Autodesk Fusion 360 part; units mm, degrees
(part 2 of 40)
  line L405 (261.8534, 192.3041) -> (262.0044, 192.3574) construction
  line L406 (262.0044, 192.3574) -> (262.156, 192.4097) construction
  line L407 (262.156, 192.4097) -> (262.3081, 192.461) construction
  line L408 (262.3081, 192.461) -> (262.4608, 192.5114) construction
  line L409 (262.4608, 192.5114) -> (262.614, 192.5608) construction
  line L410 (262.614, 192.5608) -> (262.7678, 192.6094) construction
  line L411 (262.7678, 192.6094) -> (262.922, 192.657) construction
  line L412 (262.922, 192.657) -> (263.0767, 192.7037) construction
  line L413 (263.0767, 192.7037) -> (263.2319, 192.7495) construction
  line L414 (263.2319, 192.7495) -> (263.3876, 192.7945) construction
  line L415 (263.3876, 192.7945) -> (263.5438, 192.8386) construction
  line L416 (263.5438, 192.8386) -> (263.7004, 192.8818) construction
  line L417 (263.7004, 192.8818) -> (263.8575, 192.9241) construction
  line L418 (263.8575, 192.9241) -> (264.015, 192.9656) construction
  line L419 (264.015, 192.9656) -> (264.1729, 193.0063) construction
  line L420 (264.1729, 193.0063) -> (264.3313, 193.0461) construction
  line L421 (264.3313, 193.0461) -> (264.4901, 193.085) construction
  line L422 (264.4901, 193.085) -> (264.6493, 193.1231) construction
  line L423 (264.6493, 193.1231) -> (264.8089, 193.1604) construction
  line L424 (264.8089, 193.1604) -> (264.9689, 193.1969) construction
  line L425 (264.9689, 193.1969) -> (265.1293, 193.2326) construction
  line L426 (265.1293, 193.2326) -> (265.2901, 193.2674) construction
  line L427 (265.2901, 193.2674) -> (265.4513, 193.3015) construction
  line L428 (265.4513, 193.3015) -> (265.6129, 193.3347) construction
  line L429 (265.6129, 193.3347) -> (265.7748, 193.3672) construction
  line L430 (265.7748, 193.3672) -> (265.9371, 193.3988) construction
  line L431 (265.9371, 193.3988) -> (266.0997, 193.4297) construction
  line L432 (266.0997, 193.4297) -> (266.2627, 193.4597) construction
  line L433 (266.2627, 193.4597) -> (266.426, 193.489) construction
  line L434 (266.426, 193.489) -> (266.5897, 193.5175) construction
  line L435 (266.5897, 193.5175) -> (266.7537, 193.5453) construction
  line L436 (266.7537, 193.5453) -> (266.9181, 193.5723) construction
  line L437 (266.9181, 193.5723) -> (267.0828, 193.5984) construction
  line L438 (267.0828, 193.5984) -> (267.2478, 193.6239) construction
  line L439 (267.2478, 193.6239) -> (267.4131, 193.6486) construction
  line L440 (267.4131, 193.6486) -> (267.5787, 193.6725) construction
  line L441 (267.5787, 193.6725) -> (267.7446, 193.6956) construction
  line L442 (267.7446, 193.6956) -> (267.9109, 193.718) construction
  line L443 (267.9109, 193.718) -> (268.0774, 193.7397) construction
  line L444 (268.0774, 193.7397) -> (268.2442, 193.7606) construction
  line L445 (268.2442, 193.7606) -> (268.3779, 193.7767) construction
  line L446 (268.3779, 193.7767) -> (268.4783, 193.7885) construction
  line L447 (268.4783, 193.7885) -> (268.5453, 193.7962) construction
  line L448 (268.5453, 193.7962) -> (268.5789, 193.8) construction
  arc A3 (253.9452, 189.3784) -> (251.5104, 191.8132) centre (212.132, 150) ccw
  line L449 (256.7226, 189.2483) -> (257.9473, 190.3263)
  arc A4 (253.9452, 189.3784) -> (256.7226, 189.2483) centre (255.4012, 190.7496) ccw
  spline S6 degree 5 poles (252.4583, 195.8153) (252.4787, 195.8385) (252.5188, 195.8854) (252.5771, 195.9573) (252.6512, 196.056) (252.7386, 196.1833) (252.8224, 196.3135) (252.904, 196.4454) (252.9844, 196.5782) (253.064, 196.7117) (253.1427, 196.8458) (253.2203, 196.9807) (253.2962, 197.1168) (253.3703, 197.2543) (253.4426, 197.393) (253.5133, 197.5329) (253.5824, 197.6738) (253.6504, 197.8156) (253.7173, 197.9581) (253.7832, 198.1012) (253.848, 198.245) (253.9118, 198.3895) (253.9744, 198.5347) (254.0359, 198.6807) (254.0962, 198.8274) (254.1554, 198.9749) (254.2135, 199.123) (254.2706, 199.2717) (254.3267, 199.421) (254.3819, 199.5709) (254.4361, 199.7214) (254.4894, 199.8724) (254.5417, 200.024) (254.593, 200.1761) (254.6434, 200.3288) (254.6928, 200.482) (254.7414, 200.6358) (254.789, 200.79) (254.8357, 200.9447) (254.8815, 201.0999) (254.9265, 201.2556) (254.9706, 201.4118) (255.0138, 201.5684) (255.0561, 201.7255) (255.0976, 201.883) (255.1383, 202.0409) (255.1781, 202.1993) (255.217, 202.3581) (255.2551, 202.5173) (255.2924, 202.6769) (255.3289, 202.8369) (255.3646, 202.9973) (255.3994, 203.1581) (255.4335, 203.3193) (255.4667, 203.4809) (255.4992, 203.6428) (255.5308, 203.8051) (255.5617, 203.9677) (255.5917, 204.1307) (255.621, 204.294) (255.6495, 204.4577) (255.6773, 204.6217) (255.7043, 204.7861) (255.7304, 204.9508) (255.7559, 205.1158) (255.7806, 205.2811) (255.8045, 205.4467) (255.8276, 205.6126) (255.85, 205.7789) (255.8717, 205.9454) (255.8926, 206.1122) (255.9087, 206.2459) (255.9205, 206.3463) (255.9282, 206.4133) (255.932, 206.4469) knots 0 0 0 0 0 0 0.01428571 0.02857143 0.04285714 0.05714286 0.07142857 0.08571429 0.1 0.11428571 0.12857143 0.14285714 0.15714286 0.17142857 0.18571429 0.2 0.21428571 0.22857143 0.24285714 0.25714286 0.27142857 0.28571429 0.3 0.31428571 0.32857143 0.34285714 0.35714286 0.37142857 0.38571429 0.4 0.41428571 0.42857143 0.44285714 0.45714286 0.47142857 0.48571429 0.5 0.51428571 0.52857143 0.54285714 0.55714286 0.57142857 0.58571429 0.6 0.61428571 0.62857143 0.64285714 0.65714286 0.67142857 0.68571429 0.7 0.71428571 0.72857143 0.74285714 0.75714286 0.77142857 0.78571429 0.8 0.81428571 0.82857143 0.84285714 0.85714286 0.87142857 0.88571429 0.9 0.91428571 0.92857143 0.94285714 0.95714286 0.97142857 0.98571429 1 1 1 1 1 1
  line L450 (252.4583, 195.8153) -> (252.4787, 195.8385) construction
  line L451 (252.4787, 195.8385) -> (252.5188, 195.8854) construction
  line L452 (252.5188, 195.8854) -> (252.5771, 195.9573) construction
  line L453 (252.5771, 195.9573) -> (252.6512, 196.056) construction
  line L454 (252.6512, 196.056) -> (252.7386, 196.1833) construction
  line L455 (252.7386, 196.1833) -> (252.8224, 196.3135) construction
  line L456 (252.8224, 196.3135) -> (252.904, 196.4454) construction
  line L457 (252.904, 196.4454) -> (252.9844, 196.5782) construction
  line L458 (252.9844, 196.5782) -> (253.064, 196.7117) construction
  line L459 (253.064, 196.7117) -> (253.1427, 196.8458) construction
  line L460 (253.1427, 196.8458) -> (253.2203, 196.9807) construction
  line L461 (253.2203, 196.9807) -> (253.2962, 197.1168) construction
  line L462 (253.2962, 197.1168) -> (253.3703, 197.2543) construction
  line L463 (253.3703, 197.2543) -> (253.4426, 197.393) construction
  line L464 (253.4426, 197.393) -> (253.5133, 197.5329) construction
  line L465 (253.5133, 197.5329) -> (253.5824, 197.6738) construction
  line L466 (253.5824, 197.6738) -> (253.6504, 197.8156) construction
  line L467 (253.6504, 197.8156) -> (253.7173, 197.9581) construction
  line L468 (253.7173, 197.9581) -> (253.7832, 198.1012) construction
  line L469 (253.7832, 198.1012) -> (253.848, 198.245) construction
  line L470 (253.848, 198.245) -> (253.9118, 198.3895) construction
  line L471 (253.9118, 198.3895) -> (253.9744, 198.5347) construction
  line L472 (253.9744, 198.5347) -> (254.0359, 198.6807) construction
  line L473 (254.0359, 198.6807) -> (254.0962, 198.8274) construction
  line L474 (254.0962, 198.8274) -> (254.1554, 198.9749) construction
  line L475 (254.1554, 198.9749) -> (254.2135, 199.123) construction
  line L476 (254.2135, 199.123) -> (254.2706, 199.2717) construction
  line L477 (254.2706, 199.2717) -> (254.3267, 199.421) construction
  line L478 (254.3267, 199.421) -> (254.3819, 199.5709) construction
  line L479 (254.3819, 199.5709) -> (254.4361, 199.7214) construction
  line L480 (254.4361, 199.7214) -> (254.4894, 199.8724) construction
  line L481 (254.4894, 199.8724) -> (254.5417, 200.024) construction
  line L482 (254.5417, 200.024) -> (254.593, 200.1761) construction
  line L483 (254.593, 200.1761) -> (254.6434, 200.3288) construction
  line L484 (254.6434, 200.3288) -> (254.6928, 200.482) construction
  line L485 (254.6928, 200.482) -> (254.7414, 200.6358) construction
  line L486 (254.7414, 200.6358) -> (254.789, 200.79) construction
  line L487 (254.789, 200.79) -> (254.8357, 200.9447) construction
  line L488 (254.8357, 200.9447) -> (254.8815, 201.0999) construction
  line L489 (254.8815, 201.0999) -> (254.9265, 201.2556) construction
  line L490 (254.9265, 201.2556) -> (254.9706, 201.4118) construction
  line L491 (254.9706, 201.4118) -> (255.0138, 201.5684) construction
  line L492 (255.0138, 201.5684) -> (255.0561, 201.7255) construction
  line L493 (255.0561, 201.7255) -> (255.0976, 201.883) construction
  line L494 (255.0976, 201.883) -> (255.1383, 202.0409) construction
  line L495 (255.1383, 202.0409) -> (255.1781, 202.1993) construction
  line L496 (255.1781, 202.1993) -> (255.217, 202.3581) construction
  line L497 (255.217, 202.3581) -> (255.2551, 202.5173) construction
  line L498 (255.2551, 202.5173) -> (255.2924, 202.6769) construction
  line L499 (255.2924, 202.6769) -> (255.3289, 202.8369) construction
  line L500 (255.3289, 202.8369) -> (255.3646, 202.9973) construction
  line L501 (255.3646, 202.9973) -> (255.3994, 203.1581) construction
  line L502 (255.3994, 203.1581) -> (255.4335, 203.3193) construction
  line L503 (255.4335, 203.3193) -> (255.4667, 203.4809) construction
  line L504 (255.4667, 203.4809) -> (255.4992, 203.6428) construction
  line L505 (255.4992, 203.6428) -> (255.5308, 203.8051) construction
  line L506 (255.5308, 203.8051) -> (255.5617, 203.9677) construction
  line L507 (255.5617, 203.9677) -> (255.5917, 204.1307) construction
  line L508 (255.5917, 204.1307) -> (255.621, 204.294) construction
  line L509 (255.621, 204.294) -> (255.6495, 204.4577) construction
  line L510 (255.6495, 204.4577) -> (255.6773, 204.6217) construction
  line L511 (255.6773, 204.6217) -> (255.7043, 204.7861) construction
  line L512 (255.7043, 204.7861) -> (255.7304, 204.9508) construction
  line L513 (255.7304, 204.9508) -> (255.7559, 205.1158) construction
  line L514 (255.7559, 205.1158) -> (255.7806, 205.2811) construction
  line L515 (255.7806, 205.2811) -> (255.8045, 205.4467) construction
  line L516 (255.8045, 205.4467) -> (255.8276, 205.6126) construction
  line L517 (255.8276, 205.6126) -> (255.85, 205.7789) construction
  line L518 (255.85, 205.7789) -> (255.8717, 205.9454) construction
  line L519 (255.8717, 205.9454) -> (255.8926, 206.1122) construction
  line L520 (255.8926, 206.1122) -> (255.9087, 206.2459) construction
  line L521 (255.9087, 206.2459) -> (255.9205, 206.3463) construction
  line L522 (255.9205, 206.3463) -> (255.9282, 206.4133) construction
  line L523 (255.9282, 206.4133) -> (255.932, 206.4469) construction
  arc A5 (271.2313, 190.1492) -> (268.5789, 193.8) centre (212.132, 150) ccw
  arc A6 (271.2313, 190.1492) -> (268.5789, 193.8) centre (212.132, 150) ccw
  spline S7 degree 5 poles (252.4583, 195.8153) (252.4787, 195.8385) (252.5188, 195.8854) (252.5771, 195.9573) (252.6512, 196.056) (252.7386, 196.1833) (252.8224, 196.3135) (252.904, 196.4454) (252.9844, 196.5782) (253.064, 196.7117) (253.1427, 196.8458) (253.2203, 196.9807) (253.2962, 197.1168) (253.3703, 197.2543) (253.4426, 197.393) (253.5133, 197.5329) (253.5824, 197.6738) (253.6504, 197.8156) (253.7173, 197.9581) (253.7832, 198.1012) (253.848, 198.245) (253.9118, 198.3895) (253.9744, 198.5347) (254.0359, 198.6807) (254.0962, 198.8274) (254.1554, 198.9749) (254.2135, 199.123) (254.2706, 199.2717) (254.3267, 199.421) (254.3819, 199.5709) (254.4361, 199.7214) (254.4894, 199.8724) (254.5417, 200.024) (254.593, 200.1761) (254.6434, 200.3288) (254.6928, 200.482) (254.7414, 200.6358) (254.789, 200.79) (254.8357, 200.9447) (254.8815, 201.0999) (254.9265, 201.2556) (254.9706, 201.4118) (255.0138, 201.5684) (255.0561, 201.7255) (255.0976, 201.883) (255.1383, 202.0409) (255.1781, 202.1993) (255.217, 202.3581) (255.2551, 202.5173) (255.2924, 202.6769) (255.3289, 202.8369) (255.3646, 202.9973) (255.3994, 203.1581) (255.4335, 203.3193) (255.4667, 203.4809) (255.4992, 203.6428) (255.5308, 203.8051) (255.5617, 203.9677) (255.5917, 204.1307) (255.621, 204.294) (255.6495, 204.4577) (255.6773, 204.6217) (255.7043, 204.7861) (255.7304, 204.9508) (255.7559, 205.1158) (255.7806, 205.2811) (255.8045, 205.4467) (255.8276, 205.6126) (255.85, 205.7789) (255.8717, 205.9454) (255.8926, 206.1122) (255.9087, 206.2459) (255.9205, 206.3463) (255.9282, 206.4133) (255.932, 206.4469) knots 0 0 0 0 0 0 0.01428571 0.02857143 0.04285714 0.05714286 0.07142857 0.08571429 0.1 0.11428571 0.12857143 0.14285714 0.15714286 0.17142857 0.18571429 0.2 0.21428571 0.22857143 0.24285714 0.25714286 0.27142857 0.28571429 0.3 0.31428571 0.32857143 0.34285714 0.35714286 0.37142857 0.38571429 0.4 0.41428571 0.42857143 0.44285714 0.45714286 0.47142857 0.48571429 0.5 0.51428571 0.52857143 0.54285714 0.55714286 0.57142857 0.58571429 0.6 0.61428571 0.62857143 0.64285714 0.65714286 0.67142857 0.68571429 0.7 0.71428571 0.72857143 0.74285714 0.75714286 0.77142857 0.78571429 0.8 0.81428571 0.82857143 0.84285714 0.85714286 0.87142857 0.88571429 0.9 0.91428571 0.92857143 0.94285714 0.95714286 0.97142857 0.98571429 1 1 1 1 1 1
  line L524 (252.4583, 195.8153) -> (252.4787, 195.8385) construction
  line L525 (252.4787, 195.8385) -> (252.5188, 195.8854) construction
  line L526 (252.5188, 195.8854) -> (252.5771, 195.9573) construction
  line L527 (252.5771, 195.9573) -> (252.6512, 196.056) construction
  line L528 (252.6512, 196.056) -> (252.7386, 196.1833) construction
  line L529 (252.7386, 196.1833) -> (252.8224, 196.3135) construction
  line L530 (252.8224, 196.3135) -> (252.904, 196.4454) construction
  line L531 (252.904, 196.4454) -> (252.9844, 196.5782) construction
  line L532 (252.9844, 196.5782) -> (253.064, 196.7117) construction
  line L533 (253.064, 196.7117) -> (253.1427, 196.8458) construction
  line L534 (253.1427, 196.8458) -> (253.2203, 196.9807) construction
  line L535 (253.2203, 196.9807) -> (253.2962, 197.1168) construction
  line L536 (253.2962, 197.1168) -> (253.3703, 197.2543) construction
  line L537 (253.3703, 197.2543) -> (253.4426, 197.393) construction
  line L538 (253.4426, 197.393) -> (253.5133, 197.5329) construction
  line L539 (253.5133, 197.5329) -> (253.5824, 197.6738) construction
  line L540 (253.5824, 197.6738) -> (253.6504, 197.8156) construction
  line L541 (253.6504, 197.8156) -> (253.7173, 197.9581) construction
  line L542 (253.7173, 197.9581) -> (253.7832, 198.1012) construction
  line L543 (253.7832, 198.1012) -> (253.848, 198.245) construction
  line L544 (253.848, 198.245) -> (253.9118, 198.3895) construction
  line L545 (253.9118, 198.3895) -> (253.9744, 198.5347) construction
  line L546 (253.9744, 198.5347) -> (254.0359, 198.6807) construction
  line L547 (254.0359, 198.6807) -> (254.0962, 198.8274) construction
  line L548 (254.0962, 198.8274) -> (254.1554, 198.9749) construction
  line L549 (254.1554, 198.9749) -> (254.2135, 199.123) construction
  line L550 (254.2135, 199.123) -> (254.2706, 199.2717) construction
  line L551 (254.2706, 199.2717) -> (254.3267, 199.421) construction
  line L552 (254.3267, 199.421) -> (254.3819, 199.5709) construction
  line L553 (254.3819, 199.5709) -> (254.4361, 199.7214) construction
  line L554 (254.4361, 199.7214) -> (254.4894, 199.8724) construction
  line L555 (254.4894, 199.8724) -> (254.5417, 200.024) construction
  line L556 (254.5417, 200.024) -> (254.593, 200.1761) construction
  line L557 (254.593, 200.1761) -> (254.6434, 200.3288) construction
  line L558 (254.6434, 200.3288) -> (254.6928, 200.482) construction
  line L559 (254.6928, 200.482) -> (254.7414, 200.6358) construction
  line L560 (254.7414, 200.6358) -> (254.789, 200.79) construction
  line L561 (254.789, 200.79) -> (254.8357, 200.9447) construction
  line L562 (254.8357, 200.9447) -> (254.8815, 201.0999) construction
  line L563 (254.8815, 201.0999) -> (254.9265, 201.2556) construction
  line L564 (254.9265, 201.2556) -> (254.9706, 201.4118) construction
  line L565 (254.9706, 201.4118) -> (255.0138, 201.5684) construction
  line L566 (255.0138, 201.5684) -> (255.0561, 201.7255) construction
  line L567 (255.0561, 201.7255) -> (255.0976, 201.883) construction
  line L568 (255.0976, 201.883) -> (255.1383, 202.0409) construction
  line L569 (255.1383, 202.0409) -> (255.1781, 202.1993) construction
  line L570 (255.1781, 202.1993) -> (255.217, 202.3581) construction
  line L571 (255.217, 202.3581) -> (255.2551, 202.5173) construction
  line L572 (255.2551, 202.5173) -> (255.2924, 202.6769) construction
  line L573 (255.2924, 202.6769) -> (255.3289, 202.8369) construction
  line L574 (255.3289, 202.8369) -> (255.3646, 202.9973) construction
  line L575 (255.3646, 202.9973) -> (255.3994, 203.1581) construction
  line L576 (255.3994, 203.1581) -> (255.4335, 203.3193) construction
  line L577 (255.4335, 203.3193) -> (255.4667, 203.4809) construction
  line L578 (255.4667, 203.4809) -> (255.4992, 203.6428) construction
  line L579 (255.4992, 203.6428) -> (255.5308, 203.8051) construction
  line L580 (255.5308, 203.8051) -> (255.5617, 203.9677) construction
  line L581 (255.5617, 203.9677) -> (255.5917, 204.1307) construction
  line L582 (255.5917, 204.1307) -> (255.621, 204.294) construction
  line L583 (255.621, 204.294) -> (255.6495, 204.4577) construction
  line L584 (255.6495, 204.4577) -> (255.6773, 204.6217) construction
  line L585 (255.6773, 204.6217) -> (255.7043, 204.7861) construction
  line L586 (255.7043, 204.7861) -> (255.7304, 204.9508) construction
  line L587 (255.7304, 204.9508) -> (255.7559, 205.1158) construction
  line L588 (255.7559, 205.1158) -> (255.7806, 205.2811) construction
  line L589 (255.7806, 205.2811) -> (255.8045, 205.4467) construction
  line L590 (255.8045, 205.4467) -> (255.8276, 205.6126) construction
  line L591 (255.8276, 205.6126) -> (255.85, 205.7789) construction
  line L592 (255.85, 205.7789) -> (255.8717, 205.9454) construction
  line L593 (255.8717, 205.9454) -> (255.8926, 206.1122) construction
  line L594 (255.8926, 206.1122) -> (255.9087, 206.2459) construction
  line L595 (255.9087, 206.2459) -> (255.9205, 206.3463) construction
  line L596 (255.9205, 206.3463) -> (255.9282, 206.4133) construction
  line L597 (255.9282, 206.4133) -> (255.932, 206.4469) construction
  spline S8 degree 5 poles (156.0975, 174.1948) (156.0692, 174.2071) (156.0122, 174.2308) (155.9258, 174.264) (155.8091, 174.3039) (155.6609, 174.3478) (155.5112, 174.3873) (155.3606, 174.4241) (155.2094, 174.4595) (155.0579, 174.494) (154.906, 174.5274) (154.7537, 174.5594) (154.6008, 174.5896) (154.4472, 174.6176) (154.2929, 174.6435) (154.138, 174.6674) (153.9826, 174.6897) (153.8268, 174.7105) (153.6706, 174.7301) (153.5141, 174.7485) (153.3573, 174.7658) (153.2002, 174.7818) (153.0427, 174.7965) (152.8849, 174.8098) (152.7267, 174.8218) (152.5682, 174.8325) (152.4094, 174.842) (152.2503, 174.8504) (152.0909, 174.8577) (151.9313, 174.8638) (151.7715, 174.8689) (151.6114, 174.8729) (151.4511, 174.8757) (151.2905, 174.8776) (151.1297, 174.8783) (150.9687, 174.878) (150.8075, 174.8766) (150.6461, 174.8742) (150.4845, 174.8708) (150.3227, 174.8665) (150.1608, 174.8611) (149.9986, 174.8548) (149.8363, 174.8475) (149.6739, 174.8392) (149.5113, 174.83) (149.3485, 174.8199) (149.1856, 174.8088) (149.0225, 174.7967) (148.8593, 174.7838) (148.696, 174.77) (148.5325, 174.7552) (148.3689, 174.7396) (148.2052, 174.723) (148.0414, 174.7056) (147.8775, 174.6873) (147.7135, 174.6681) (147.5494, 174.648) (147.3852, 174.6271) (147.2209, 174.6054) (147.0565, 174.5828) (146.892, 174.5593) (146.7274, 174.535) (146.5628, 174.5098) (146.398, 174.4839) (146.2333, 174.4571) (146.0684, 174.4294) (145.9035, 174.401) (145.7385, 174.3718) (145.5735, 174.3417) (145.4084, 174.3108) (145.2433, 174.2792) (145.1112, 174.2532) (145.0121, 174.2334) (144.946, 174.22) (144.9129, 174.2132) knots 0 0 0 0 0 0 0.01428571 0.02857143 0.04285714 0.05714286 0.07142857 0.08571429 0.1 0.11428571 0.12857143 0.14285714 0.15714286 0.17142857 0.18571429 0.2 0.21428571 0.22857143 0.24285714 0.25714286 0.27142857 0.28571429 0.3 0.31428571 0.32857143 0.34285714 0.35714286 0.37142857 0.38571429 0.4 0.41428571 0.42857143 0.44285714 0.45714286 0.47142857 0.48571429 0.5 0.51428571 0.52857143 0.54285714 0.55714286 0.57142857 0.58571429 0.6 0.61428571 0.62857143 0.64285714 0.65714286 0.67142857 0.68571429 0.7 0.71428571 0.72857143 0.74285714 0.75714286 0.77142857 0.78571429 0.8 0.81428571 0.82857143 0.84285714 0.85714286 0.87142857 0.88571429 0.9 0.91428571 0.92857143 0.94285714 0.95714286 0.97142857 0.98571429 1 1 1 1 1 1
  line L598 (156.0975, 174.1948) -> (156.0692, 174.2071) construction
  line L599 (156.0692, 174.2071) -> (156.0122, 174.2308) construction
  line L600 (156.0122, 174.2308) -> (155.9258, 174.264) construction
  line L601 (155.9258, 174.264) -> (155.8091, 174.3039) construction
  line L602 (155.8091, 174.3039) -> (155.6609, 174.3478) construction
  line L603 (155.6609, 174.3478) -> (155.5112, 174.3873) construction
  line L604 (155.5112, 174.3873) -> (155.3606, 174.4241) construction
  line L605 (155.3606, 174.4241) -> (155.2094, 174.4595) construction
  line L606 (155.2094, 174.4595) -> (155.0579, 174.494) construction
  line L607 (155.0579, 174.494) -> (154.906, 174.5274) construction
  line L608 (154.906, 174.5274) -> (154.7537, 174.5594) construction
  line L609 (154.7537, 174.5594) -> (154.6008, 174.5896) construction
  line L610 (154.6008, 174.5896) -> (154.4472, 174.6176) construction
  line L611 (154.4472, 174.6176) -> (154.2929, 174.6435) construction
  line L612 (154.2929, 174.6435) -> (154.138, 174.6674) construction
  line L613 (154.138, 174.6674) -> (153.9826, 174.6897) construction
  line L614 (153.9826, 174.6897) -> (153.8268, 174.7105) construction
  line L615 (153.8268, 174.7105) -> (153.6706, 174.7301) construction
  line L616 (153.6706, 174.7301) -> (153.5141, 174.7485) construction
  line L617 (153.5141, 174.7485) -> (153.3573, 174.7658) construction
  line L618 (153.3573, 174.7658) -> (153.2002, 174.7818) construction
  line L619 (153.2002, 174.7818) -> (153.0427, 174.7965) construction
  line L620 (153.0427, 174.7965) -> (152.8849, 174.8098) construction
  line L621 (152.8849, 174.8098) -> (152.7267, 174.8218) construction
  line L622 (152.7267, 174.8218) -> (152.5682, 174.8325) construction
  line L623 (152.5682, 174.8325) -> (152.4094, 174.842) construction
  line L624 (152.4094, 174.842) -> (152.2503, 174.8504) construction
  line L625 (152.2503, 174.8504) -> (152.0909, 174.8577) construction
  line L626 (152.0909, 174.8577) -> (151.9313, 174.8638) construction
  line L627 (151.9313, 174.8638) -> (151.7715, 174.8689) construction
  line L628 (151.7715, 174.8689) -> (151.6114, 174.8729) construction
  line L629 (151.6114, 174.8729) -> (151.4511, 174.8757) construction
  line L630 (151.4511, 174.8757) -> (151.2905, 174.8776) construction
  line L631 (151.2905, 174.8776) -> (151.1297, 174.8783) construction
  line L632 (151.1297, 174.8783) -> (150.9687, 174.878) construction
  line L633 (150.9687, 174.878) -> (150.8075, 174.8766) construction
  line L634 (150.8075, 174.8766) -> (150.6461, 174.8742) construction
  line L635 (150.6461, 174.8742) -> (150.4845, 174.8708) construction
  line L636 (150.4845, 174.8708) -> (150.3227, 174.8665) construction
  line L637 (150.3227, 174.8665) -> (150.1608, 174.8611) construction
  line L638 (150.1608, 174.8611) -> (149.9986, 174.8548) construction
  line L639 (149.9986, 174.8548) -> (149.8363, 174.8475) construction
  line L640 (149.8363, 174.8475) -> (149.6739, 174.8392) construction
  line L641 (149.6739, 174.8392) -> (149.5113, 174.83) construction
  line L642 (149.5113, 174.83) -> (149.3485, 174.8199) construction
  line L643 (149.3485, 174.8199) -> (149.1856, 174.8088) construction
  line L644 (149.1856, 174.8088) -> (149.0225, 174.7967) construction
  line L645 (149.0225, 174.7967) -> (148.8593, 174.7838) construction
  line L646 (148.8593, 174.7838) -> (148.696, 174.77) construction
  line L647 (148.696, 174.77) -> (148.5325, 174.7552) construction
  line L648 (148.5325, 174.7552) -> (148.3689, 174.7396) construction
  line L649 (148.3689, 174.7396) -> (148.2052, 174.723) construction
  line L650 (148.2052, 174.723) -> (148.0414, 174.7056) construction
  line L651 (148.0414, 174.7056) -> (147.8775, 174.6873) construction
  line L652 (147.8775, 174.6873) -> (147.7135, 174.6681) construction
  line L653 (147.7135, 174.6681) -> (147.5494, 174.648) construction
  line L654 (147.5494, 174.648) -> (147.3852, 174.6271) construction
  line L655 (147.3852, 174.6271) -> (147.2209, 174.6054) construction
  line L656 (147.2209, 174.6054) -> (147.0565, 174.5828) construction
  line L657 (147.0565, 174.5828) -> (146.892, 174.5593) construction
  line L658 (146.892, 174.5593) -> (146.7274, 174.535) construction
  line L659 (146.7274, 174.535) -> (146.5628, 174.5098) construction
  line L660 (146.5628, 174.5098) -> (146.398, 174.4839) construction
  line L661 (146.398, 174.4839) -> (146.2333, 174.4571) construction
  line L662 (146.2333, 174.4571) -> (146.0684, 174.4294) construction
  line L663 (146.0684, 174.4294) -> (145.9035, 174.401) construction
  line L664 (145.9035, 174.401) -> (145.7385, 174.3718) construction
  line L665 (145.7385, 174.3718) -> (145.5735, 174.3417) construction
  line L666 (145.5735, 174.3417) -> (145.4084, 174.3108) construction
  line L667 (145.4084, 174.3108) -> (145.2433, 174.2792) construction
  line L668 (145.2433, 174.2792) -> (145.1112, 174.2532) construction
  line L669 (145.1112, 174.2532) -> (145.0121, 174.2334) construction
  line L670 (145.0121, 174.2334) -> (144.946, 174.22) construction
  line L671 (144.946, 174.22) -> (144.9129, 174.2132) construction
  arc A7 (160.1966, 125.4699) -> (157.5954, 126.4519) centre (158.3882, 124.6158) ccw
  arc A8 (144.9129, 174.2132) -> (143.5184, 169.9215) centre (212.132, 150) ccw
  line L672 (157.5954, 173.5481) -> (156.0975, 174.1948)
  arc A9 (155.1583, 142.7194) -> (152.9878, 144.4572) centre (153.1745, 142.4659) ccw
  spline S9 degree 5 poles (156.0975, 125.8052) (156.0692, 125.7929) (156.0122, 125.7692) (155.9258, 125.736) (155.8091, 125.6961) (155.6609, 125.6522) (155.5112, 125.6127) (155.3606, 125.5759) (155.2094, 125.5405) (155.0579, 125.506) (154.906, 125.4726) (154.7537, 125.4406) (154.6008, 125.4104) (154.4472, 125.3824) (154.2929, 125.3565) (154.138, 125.3326) (153.9826, 125.3103) (153.8268, 125.2895) (153.6706, 125.2699) (153.5141, 125.2515) (153.3573, 125.2342) (153.2002, 125.2182) (153.0427, 125.2035) (152.8849, 125.1902) (152.7267, 125.1782) (152.5682, 125.1675) (152.4094, 125.158) (152.2503, 125.1496) (152.0909, 125.1423) (151.9313, 125.1362) (151.7715, 125.1311) (151.6114, 125.1271) (151.4511, 125.1243) (151.2905, 125.1224) (151.1297, 125.1217) (150.9687, 125.122) (150.8075, 125.1234) (150.6461, 125.1258) (150.4845, 125.1292) (150.3227, 125.1335) (150.1608, 125.1389) (149.9986, 125.1452) (149.8363, 125.1525) (149.6739, 125.1608) (149.5113, 125.17) (149.3485, 125.1801) (149.1856, 125.1912) (149.0225, 125.2033) (148.8593, 125.2162) (148.696, 125.23) (148.5325, 125.2448) (148.3689, 125.2604) (148.2052, 125.277) (148.0414, 125.2944) (147.8775, 125.3127) (147.7135, 125.3319) (147.5494, 125.352) (147.3852, 125.3729) (147.2209, 125.3946) (147.0565, 125.4172) (146.892, 125.4407) (146.7274, 125.465) (146.5628, 125.4902) (146.398, 125.5161) (146.2333, 125.5429) (146.0684, 125.5706) (145.9035, 125.599) (145.7385, 125.6282) (145.5735, 125.6583) (145.4084, 125.6892) (145.2433, 125.7208) (145.1112, 125.7468) (145.0121, 125.7666) (144.946, 125.78) (144.9129, 125.7868) knots 0 0 0 0 0 0 0.01428571 0.02857143 0.04285714 0.05714286 0.07142857 0.08571429 0.1 0.11428571 0.12857143 0.14285714 0.15714286 0.17142857 0.18571429 0.2 0.21428571 0.22857143 0.24285714 0.25714286 0.27142857 0.28571429 0.3 0.31428571 0.32857143 0.34285714 0.35714286 0.37142857 0.38571429 0.4 0.41428571 0.42857143 0.44285714 0.45714286 0.47142857 0.48571429 0.5 0.51428571 0.52857143 0.54285714 0.55714286 0.57142857 0.58571429 0.6 0.61428571 0.62857143 0.64285714 0.65714286 0.67142857 0.68571429 0.7 0.71428571 0.72857143 0.74285714 0.75714286 0.77142857 0.78571429 0.8 0.81428571 0.82857143 0.84285714 0.85714286 0.87142857 0.88571429 0.9 0.91428571 0.92857143 0.94285714 0.95714286 0.97142857 0.98571429 1 1 1 1 1 1
  line L673 (156.0975, 125.8052) -> (156.0692, 125.7929) construction
  line L674 (156.0692, 125.7929) -> (156.0122, 125.7692) construction
  line L675 (156.0122, 125.7692) -> (155.9258, 125.736) construction
  line L676 (155.9258, 125.736) -> (155.8091, 125.6961) construction
  line L677 (155.8091, 125.6961) -> (155.6609, 125.6522) construction
  line L678 (155.6609, 125.6522) -> (155.5112, 125.6127) construction
  line L679 (155.5112, 125.6127) -> (155.3606, 125.5759) construction
  line L680 (155.3606, 125.5759) -> (155.2094, 125.5405) construction
  line L681 (155.2094, 125.5405) -> (155.0579, 125.506) construction
  line L682 (155.0579, 125.506) -> (154.906, 125.4726) construction
  line L683 (154.906, 125.4726) -> (154.7537, 125.4406) construction
  line L684 (154.7537, 125.4406) -> (154.6008, 125.4104) construction
  line L685 (154.6008, 125.4104) -> (154.4472, 125.3824) construction
  line L686 (154.4472, 125.3824) -> (154.2929, 125.3565) construction
  line L687 (154.2929, 125.3565) -> (154.138, 125.3326) construction
  line L688 (154.138, 125.3326) -> (153.9826, 125.3103) construction
  line L689 (153.9826, 125.3103) -> (153.8268, 125.2895) construction
  line L690 (153.8268, 125.2895) -> (153.6706, 125.2699) construction
  line L691 (153.6706, 125.2699) -> (153.5141, 125.2515) construction
  line L692 (153.5141, 125.2515) -> (153.3573, 125.2342) construction
  line L693 (153.3573, 125.2342) -> (153.2002, 125.2182) construction
  line L694 (153.2002, 125.2182) -> (153.0427, 125.2035) construction
  line L695 (153.0427, 125.2035) -> (152.8849, 125.1902) construction
  line L696 (152.8849, 125.1902) -> (152.7267, 125.1782) construction
  line L697 (152.7267, 125.1782) -> (152.5682, 125.1675) construction
  line L698 (152.5682, 125.1675) -> (152.4094, 125.158) construction
  line L699 (152.4094, 125.158) -> (152.2503, 125.1496) construction
  line L700 (152.2503, 125.1496) -> (152.0909, 125.1423) construction
  line L701 (152.0909, 125.1423) -> (151.9313, 125.1362) construction
  line L702 (151.9313, 125.1362) -> (151.7715, 125.1311) construction
  line L703 (151.7715, 125.1311) -> (151.6114, 125.1271) construction
  line L704 (151.6114, 125.1271) -> (151.4511, 125.1243) construction
  line L705 (151.4511, 125.1243) -> (151.2905, 125.1224) construction
  line L706 (151.2905, 125.1224) -> (151.1297, 125.1217) construction
  line L707 (151.1297, 125.1217) -> (150.9687, 125.122) construction
  line L708 (150.9687, 125.122) -> (150.8075, 125.1234) construction
  line L709 (150.8075, 125.1234) -> (150.6461, 125.1258) construction
  line L710 (150.6461, 125.1258) -> (150.4845, 125.1292) construction
  line L711 (150.4845, 125.1292) -> (150.3227, 125.1335) construction
  line L712 (150.3227, 125.1335) -> (150.1608, 125.1389) construction
  line L713 (150.1608, 125.1389) -> (149.9986, 125.1452) construction
  line L714 (149.9986, 125.1452) -> (149.8363, 125.1525) construction
  line L715 (149.8363, 125.1525) -> (149.6739, 125.1608) construction
  line L716 (149.6739, 125.1608) -> (149.5113, 125.17) construction
  line L717 (149.5113, 125.17) -> (149.3485, 125.1801) construction
  line L718 (149.3485, 125.1801) -> (149.1856, 125.1912) construction
  line L719 (149.1856, 125.1912) -> (149.0225, 125.2033) construction
  line L720 (149.0225, 125.2033) -> (148.8593, 125.2162) construction
  line L721 (148.8593, 125.2162) -> (148.696, 125.23) construction
  line L722 (148.696, 125.23) -> (148.5325, 125.2448) construction
  line L723 (148.5325, 125.2448) -> (148.3689, 125.2604) construction
  line L724 (148.3689, 125.2604) -> (148.2052, 125.277) construction
  line L725 (148.2052, 125.277) -> (148.0414, 125.2944) construction
  line L726 (148.0414, 125.2944) -> (147.8775, 125.3127) construction
  line L727 (147.8775, 125.3127) -> (147.7135, 125.3319) construction
  line L728 (147.7135, 125.3319) -> (147.5494, 125.352) construction
  line L729 (147.5494, 125.352) -> (147.3852, 125.3729) construction
  line L730 (147.3852, 125.3729) -> (147.2209, 125.3946) construction
  line L731 (147.2209, 125.3946) -> (147.0565, 125.4172) construction
  line L732 (147.0565, 125.4172) -> (146.892, 125.4407) construction
  line L733 (146.892, 125.4407) -> (146.7274, 125.465) construction
  line L734 (146.7274, 125.465) -> (146.5628, 125.4902) construction
  line L735 (146.5628, 125.4902) -> (146.398, 125.5161) construction
  line L736 (146.398, 125.5161) -> (146.2333, 125.5429) construction
  line L737 (146.2333, 125.5429) -> (146.0684, 125.5706) construction
  line L738 (146.0684, 125.5706) -> (145.9035, 125.599) construction
  line L739 (145.9035, 125.599) -> (145.7385, 125.6282) construction
  line L740 (145.7385, 125.6282) -> (145.5735, 125.6583) construction
  line L741 (145.5735, 125.6583) -> (145.4084, 125.6892) construction
  line L742 (145.4084, 125.6892) -> (145.2433, 125.7208) construction
  line L743 (145.2433, 125.7208) -> (145.1112, 125.7468) construction
  line L744 (145.1112, 125.7468) -> (145.0121, 125.7666) construction
  line L745 (145.0121, 125.7666) -> (144.946, 125.78) construction
  line L746 (144.946, 125.78) -> (144.9129, 125.7868) construction
  arc A10 (140.7205, 152.2563) -> (140.7205, 147.7437) centre (212.132, 150) ccw
  spline S10 degree 5 poles (152.5778, 163.3622) (152.5477, 163.369) (152.4876, 163.3833) (152.3982, 163.4071) (152.2803, 163.4435) (152.1347, 163.4951) (151.9904, 163.5511) (151.8468, 163.6099) (151.7037, 163.6701) (151.5609, 163.7313) (151.4184, 163.7935) (151.2763, 163.8571) (151.1349, 163.9226) (150.9941, 163.9902) (150.8541, 164.06) (150.7147, 164.1316) (150.5759, 164.205) (150.4376, 164.2797) (150.2998, 164.3557) (150.1623, 164.4327) (150.0253, 164.5109) (149.8888, 164.5904) (149.7528, 164.6711) (149.6172, 164.753) (149.4822, 164.8363) (149.3477, 164.9208) (149.2136, 165.0064) (149.08, 165.0932) (148.9468, 165.181) (148.814, 165.2698) (148.6817, 165.3597) (148.5499, 165.4506) (148.4185, 165.5425) (148.2875, 165.6354) (148.157, 165.7293) (148.027, 165.8242) (147.8974, 165.92) (147.7682, 166.0168) (147.6394, 166.1146) (147.5111, 166.2132) (147.3832, 166.3127) (147.2558, 166.4131) (147.1288, 166.5144) (147.0022, 166.6166) (146.876, 166.7196) (146.7503, 166.8235) (146.625, 166.9283) (146.5002, 167.0338) (146.3758, 167.1402) (146.2518, 167.2474) (146.1282, 167.3555) (146.0051, 167.4643) (145.8823, 167.5739) (145.7601, 167.6842) (145.6382, 167.7954) (145.5168, 167.9073) (145.3958, 168.02) (145.2752, 168.1335) (145.1551, 168.2477) (145.0354, 168.3626) (144.9161, 168.4782) (144.7973, 168.5946) (144.6789, 168.7118) (144.5609, 168.8296) (144.4433, 168.9481) (144.3262, 169.0674) (144.2095, 169.1873) (144.0932, 169.3079) (143.9774, 169.4293) (143.862, 169.5512) (143.747, 169.6739) (143.6553, 169.7726) (143.5868, 169.8469) (143.5412, 169.8966) (143.5184, 169.9215) knots 0 0 0 0 0 0 0.01428571 0.02857143 0.04285714 0.05714286 0.07142857 0.08571429 0.1 0.11428571 0.12857143 0.14285714 0.15714286 0.17142857 0.18571429 0.2 0.21428571 0.22857143 0.24285714 0.25714286 0.27142857 0.28571429 0.3 0.31428571 0.32857143 0.34285714 0.35714286 0.37142857 0.38571429 0.4 0.41428571 0.42857143 0.44285714 0.45714286 0.47142857 0.48571429 0.5 0.51428571 0.52857143 0.54285714 0.55714286 0.57142857 0.58571429 0.6 0.61428571 0.62857143 0.64285714 0.65714286 0.67142857 0.68571429 0.7 0.71428571 0.72857143 0.74285714 0.75714286 0.77142857 0.78571429 0.8 0.81428571 0.82857143 0.84285714 0.85714286 0.87142857 0.88571429 0.9 0.91428571 0.92857143 0.94285714 0.95714286 0.97142857 0.98571429 1 1 1 1 1 1
  line L747 (152.5778, 163.3622) -> (152.5477, 163.369) construction
  line L748 (152.5477, 163.369) -> (152.4876, 163.3833) construction
  line L749 (152.4876, 163.3833) -> (152.3982, 163.4071) construction
  line L750 (152.3982, 163.4071) -> (152.2803, 163.4435) construction
  line L751 (152.2803, 163.4435) -> (152.1347, 163.4951) construction
  line L752 (152.1347, 163.4951) -> (151.9904, 163.5511) construction
  line L753 (151.9904, 163.5511) -> (151.8468, 163.6099) construction
  line L754 (151.8468, 163.6099) -> (151.7037, 163.6701) construction
  line L755 (151.7037, 163.6701) -> (151.5609, 163.7313) construction
  line L756 (151.5609, 163.7313) -> (151.4184, 163.7935) construction
  line L757 (151.4184, 163.7935) -> (151.2763, 163.8571) construction
  line L758 (151.2763, 163.8571) -> (151.1349, 163.9226) construction
  line L759 (151.1349, 163.9226) -> (150.9941, 163.9902) construction
  line L760 (150.9941, 163.9902) -> (150.8541, 164.06) construction
  line L761 (150.8541, 164.06) -> (150.7147, 164.1316) construction
  line L762 (150.7147, 164.1316) -> (150.5759, 164.205) construction
  line L763 (150.5759, 164.205) -> (150.4376, 164.2797) construction
  line L764 (150.4376, 164.2797) -> (150.2998, 164.3557) construction
  line L765 (150.2998, 164.3557) -> (150.1623, 164.4327) construction
  line L766 (150.1623, 164.4327) -> (150.0253, 164.5109) construction
  line L767 (150.0253, 164.5109) -> (149.8888, 164.5904) construction
  line L768 (149.8888, 164.5904) -> (149.7528, 164.6711) construction
  line L769 (149.7528, 164.6711) -> (149.6172, 164.753) construction
  line L770 (149.6172, 164.753) -> (149.4822, 164.8363) construction
  line L771 (149.4822, 164.8363) -> (149.3477, 164.9208) construction
  line L772 (149.3477, 164.9208) -> (149.2136, 165.0064) construction
  line L773 (149.2136, 165.0064) -> (149.08, 165.0932) construction
  line L774 (149.08, 165.0932) -> (148.9468, 165.181) construction
  line L775 (148.9468, 165.181) -> (148.814, 165.2698) construction
  line L776 (148.814, 165.2698) -> (148.6817, 165.3597) construction
  line L777 (148.6817, 165.3597) -> (148.5499, 165.4506) construction
  line L778 (148.5499, 165.4506) -> (148.4185, 165.5425) construction
  line L779 (148.4185, 165.5425) -> (148.2875, 165.6354) construction
  line L780 (148.2875, 165.6354) -> (148.157, 165.7293) construction
  line L781 (148.157, 165.7293) -> (148.027, 165.8242) construction
  line L782 (148.027, 165.8242) -> (147.8974, 165.92) construction
  line L783 (147.8974, 165.92) -> (147.7682, 166.0168) construction
  line L784 (147.7682, 166.0168) -> (147.6394, 166.1146) construction
  line L785 (147.6394, 166.1146) -> (147.5111, 166.2132) construction
  line L786 (147.5111, 166.2132) -> (147.3832, 166.3127) construction
  line L787 (147.3832, 166.3127) -> (147.2558, 166.4131) construction
  line L788 (147.2558, 166.4131) -> (147.1288, 166.5144) construction
  line L789 (147.1288, 166.5144) -> (147.0022, 166.6166) construction
  line L790 (147.0022, 166.6166) -> (146.876, 166.7196) construction
  line L791 (146.876, 166.7196) -> (146.7503, 166.8235) construction
  line L792 (146.7503, 166.8235) -> (146.625, 166.9283) construction
  line L793 (146.625, 166.9283) -> (146.5002, 167.0338) construction
  line L794 (146.5002, 167.0338) -> (146.3758, 167.1402) construction
  line L795 (146.3758, 167.1402) -> (146.2518, 167.2474) construction
  line L796 (146.2518, 167.2474) -> (146.1282, 167.3555) construction
  line L797 (146.1282, 167.3555) -> (146.0051, 167.4643) construction
  line L798 (146.0051, 167.4643) -> (145.8823, 167.5739) construction
  line L799 (145.8823, 167.5739) -> (145.7601, 167.6842) construction
  line L800 (145.7601, 167.6842) -> (145.6382, 167.7954) construction
  line L801 (145.6382, 167.7954) -> (145.5168, 167.9073) construction
  line L802 (145.5168, 167.9073) -> (145.3958, 168.02) construction
  line L803 (145.3958, 168.02) -> (145.2752, 168.1335) construction
  line L804 (145.2752, 168.1335) -> (145.1551, 168.2477) construction
  line L805 (145.1551, 168.2477) -> (145.0354, 168.3626) construction
  line L806 (145.0354, 168.3626) -> (144.9161, 168.4782) construction
  line L807 (144.9161, 168.4782) -> (144.7973, 168.5946) construction
  line L808 (144.7973, 168.5946) -> (144.6789, 168.7118) construction
  line L809 (144.6789, 168.7118) -> (144.5609, 168.8296) construction
  line L810 (144.5609, 168.8296) -> (144.4433, 168.9481) construction
  line L811 (144.4433, 168.9481) -> (144.3262, 169.0674) construction
  line L812 (144.3262, 169.0674) -> (144.2095, 169.1873) construction
  line L813 (144.2095, 169.1873) -> (144.0932, 169.3079) construction
  line L814 (144.0932, 169.3079) -> (143.9774, 169.4293) construction
  line L815 (143.9774, 169.4293) -> (143.862, 169.5512) construction
  line L816 (143.862, 169.5512) -> (143.747, 169.6739) construction
  line L817 (143.747, 169.6739) -> (143.6553, 169.7726) construction
  line L818 (143.6553, 169.7726) -> (143.5868, 169.8469) construction
  line L819 (143.5868, 169.8469) -> (143.5412, 169.8966) construction
  line L820 (143.5412, 169.8966) -> (143.5184, 169.9215) construction
  line L821 (157.5954, 126.4519) -> (156.0975, 125.8052)
  line L822 (161.0254, 119.7202) -> (159.6217, 118.8885)
  line L823 (152.9878, 144.4572) -> (151.3635, 144.3049)
  arc A11 (157.5954, 173.5481) -> (160.1966, 174.5301) centre (158.3882, 175.3842) ccw
  arc A12 (161.7599, 177.5982) -> (161.0254, 180.2798) centre (160.0059, 178.5592) ccw
  arc A13 (153.0327, 109.8508) -> (155.6851, 106.2) centre (212.132, 150) ccw
  arc A14 (161.0254, 119.7202) -> (161.7599, 122.4018) centre (160.0059, 121.4408) ccw
  spline S11 degree 5 poles (151.3635, 155.6951) (151.3327, 155.6979) (151.2711, 155.7029) (151.1787, 155.7078) (151.0554, 155.7097) (150.901, 155.7056) (150.7464, 155.6969) (150.5917, 155.6854) (150.437, 155.6723) (150.2822, 155.6583) (150.1275, 155.6431) (149.9727, 155.6265) (149.818, 155.608) (149.6632, 155.5871) (149.5085, 155.5641) (149.3538, 155.539) (149.1991, 155.5121) (149.0445, 155.4838) (148.8899, 155.4542) (148.7354, 155.4233) (148.5809, 155.3913) (148.4265, 155.3579) (148.2722, 155.3232) (148.118, 155.2871) (147.9638, 155.2497) (147.8098, 155.2109) (147.6558, 155.1709) (147.5019, 155.1297) (147.3481, 155.0873) (147.1944, 155.0439) (147.0408, 154.9993) (146.8873, 154.9536) (146.734, 154.9068) (146.5807, 154.8589) (146.4276, 154.8099) (146.2746, 154.7599) (146.1217, 154.7087) (145.9689, 154.6566) (145.8162, 154.6035) (145.6637, 154.5493) (145.5114, 154.4942) (145.3591, 154.438) (145.207, 154.381) (145.055, 154.3229) (144.9032, 154.2639) (144.7516, 154.2039) (144.6, 154.143) (144.4487, 154.0812) (144.2975, 154.0185) (144.1464, 153.9548) (143.9955, 153.8903) (143.8448, 153.8249) (143.6942, 153.7585) (143.5438, 153.6913) (143.3936, 153.6233) (143.2435, 153.5543) (143.0936, 153.4846) (142.9439, 153.4139) (142.7944, 153.3425) (142.645, 153.2701) (142.4958, 153.197) (142.3468, 153.123) (142.198, 153.0482) (142.0494, 152.9726) (141.9009, 152.8962) (141.7527, 152.819) (141.6046, 152.741) (141.4568, 152.6622) (141.3091, 152.5826) (141.1617, 152.5023) (141.0144, 152.4211) (140.8968, 152.3556) (140.8086, 152.3061) (140.7499, 152.2729) (140.7205, 152.2563) knots 0 0 0 0 0 0 0.01428571 0.02857143 0.04285714 0.05714286 0.07142857 0.08571429 0.1 0.11428571 0.12857143 0.14285714 0.15714286 0.17142857 0.18571429 0.2 0.21428571 0.22857143 0.24285714 0.25714286 0.27142857 0.28571429 0.3 0.31428571 0.32857143 0.34285714 0.35714286 0.37142857 0.38571429 0.4 0.41428571 0.42857143 0.44285714 0.45714286 0.47142857 0.48571429 0.5 0.51428571 0.52857143 0.54285714 0.55714286 0.57142857 0.58571429 0.6 0.61428571 0.62857143 0.64285714 0.65714286 0.67142857 0.68571429 0.7 0.71428571 0.72857143 0.74285714 0.75714286 0.77142857 0.78571429 0.8 0.81428571 0.82857143 0.84285714 0.85714286 0.87142857 0.88571429 0.9 0.91428571 0.92857143 0.94285714 0.95714286 0.97142857 0.98571429 1 1 1 1 1 1
  line L824 (151.3635, 155.6951) -> (151.3327, 155.6979) construction
  line L825 (151.3327, 155.6979) -> (151.2711, 155.7029) construction
  line L826 (151.2711, 155.7029) -> (151.1787, 155.7078) construction
  line L827 (151.1787, 155.7078) -> (151.0554, 155.7097) construction
  line L828 (151.0554, 155.7097) -> (150.901, 155.7056) construction
  line L829 (150.901, 155.7056) -> (150.7464, 155.6969) construction
  line L830 (150.7464, 155.6969) -> (150.5917, 155.6854) construction
  line L831 (150.5917, 155.6854) -> (150.437, 155.6723) construction
  line L832 (150.437, 155.6723) -> (150.2822, 155.6583) construction
  line L833 (150.2822, 155.6583) -> (150.1275, 155.6431) construction
  line L834 (150.1275, 155.6431) -> (149.9727, 155.6265) construction
  line L835 (149.9727, 155.6265) -> (149.818, 155.608) construction
  line L836 (149.818, 155.608) -> (149.6632, 155.5871) construction
  line L837 (149.6632, 155.5871) -> (149.5085, 155.5641) construction
  line L838 (149.5085, 155.5641) -> (149.3538, 155.539) construction
  line L839 (149.3538, 155.539) -> (149.1991, 155.5121) construction
  line L840 (149.1991, 155.5121) -> (149.0445, 155.4838) construction
  line L841 (149.0445, 155.4838) -> (148.8899, 155.4542) construction
  line L842 (148.8899, 155.4542) -> (148.7354, 155.4233) construction
  line L843 (148.7354, 155.4233) -> (148.5809, 155.3913) construction
  line L844 (148.5809, 155.3913) -> (148.4265, 155.3579) construction
  line L845 (148.4265, 155.3579) -> (148.2722, 155.3232) construction
  line L846 (148.2722, 155.3232) -> (148.118, 155.2871) construction
  line L847 (148.118, 155.2871) -> (147.9638, 155.2497) construction
  line L848 (147.9638, 155.2497) -> (147.8098, 155.2109) construction
  line L849 (147.8098, 155.2109) -> (147.6558, 155.1709) construction
  line L850 (147.6558, 155.1709) -> (147.5019, 155.1297) construction
  line L851 (147.5019, 155.1297) -> (147.3481, 155.0873) construction
  line L852 (147.3481, 155.0873) -> (147.1944, 155.0439) construction
  line L853 (147.1944, 155.0439) -> (147.0408, 154.9993) construction
  line L854 (147.0408, 154.9993) -> (146.8873, 154.9536) construction
  line L855 (146.8873, 154.9536) -> (146.734, 154.9068) construction
  line L856 (146.734, 154.9068) -> (146.5807, 154.8589) construction
  line L857 (146.5807, 154.8589) -> (146.4276, 154.8099) construction
  line L858 (146.4276, 154.8099) -> (146.2746, 154.7599) construction
  line L859 (146.2746, 154.7599) -> (146.1217, 154.7087) construction
  line L860 (146.1217, 154.7087) -> (145.9689, 154.6566) construction
  line L861 (145.9689, 154.6566) -> (145.8162, 154.6035) construction
  line L862 (145.8162, 154.6035) -> (145.6637, 154.5493) construction
  line L863 (145.6637, 154.5493) -> (145.5114, 154.4942) construction
  line L864 (145.5114, 154.4942) -> (145.3591, 154.438) construction
  line L865 (145.3591, 154.438) -> (145.207, 154.381) construction
  line L866 (145.207, 154.381) -> (145.055, 154.3229) construction
  line L867 (145.055, 154.3229) -> (144.9032, 154.2639) construction
  line L868 (144.9032, 154.2639) -> (144.7516, 154.2039) construction
  line L869 (144.7516, 154.2039) -> (144.6, 154.143) construction
  line L870 (144.6, 154.143) -> (144.4487, 154.0812) construction
  line L871 (144.4487, 154.0812) -> (144.2975, 154.0185) construction
  line L872 (144.2975, 154.0185) -> (144.1464, 153.9548) construction
  line L873 (144.1464, 153.9548) -> (143.9955, 153.8903) construction
  line L874 (143.9955, 153.8903) -> (143.8448, 153.8249) construction
  line L875 (143.8448, 153.8249) -> (143.6942, 153.7585) construction
  line L876 (143.6942, 153.7585) -> (143.5438, 153.6913) construction
  line L877 (143.5438, 153.6913) -> (143.3936, 153.6233) construction
  line L878 (143.3936, 153.6233) -> (143.2435, 153.5543) construction
  line L879 (143.2435, 153.5543) -> (143.0936, 153.4846) construction
  line L880 (143.0936, 153.4846) -> (142.9439, 153.4139) construction
  line L881 (142.9439, 153.4139) -> (142.7944, 153.3425) construction
  line L882 (142.7944, 153.3425) -> (142.645, 153.2701) construction
  line L883 (142.645, 153.2701) -> (142.4958, 153.197) construction
  line L884 (142.4958, 153.197) -> (142.3468, 153.123) construction
  line L885 (142.3468, 153.123) -> (142.198, 153.0482) construction
  line L886 (142.198, 153.0482) -> (142.0494, 152.9726) construction
  line L887 (142.0494, 152.9726) -> (141.9009, 152.8962) construction
  line L888 (141.9009, 152.8962) -> (141.7527, 152.819) construction
  line L889 (141.7527, 152.819) -> (141.6046, 152.741) construction
  line L890 (141.6046, 152.741) -> (141.4568, 152.6622) construction
  line L891 (141.4568, 152.6622) -> (141.3091, 152.5826) construction
  line L892 (141.3091, 152.5826) -> (141.1617, 152.5023) construction
  line L893 (141.1617, 152.5023) -> (141.0144, 152.4211) construction
  line L894 (141.0144, 152.4211) -> (140.8968, 152.3556) construction
  line L895 (140.8968, 152.3556) -> (140.8086, 152.3061) construction
  line L896 (140.8086, 152.3061) -> (140.7499, 152.2729) construction
  line L897 (140.7499, 152.2729) -> (140.7205, 152.2563) construction
  arc A15 (161.7599, 177.5982) -> (161.0254, 180.2798) centre (160.0059, 178.5592) ccw
  arc A16 (155.697, 160.6816) -> (155.1583, 157.2806) centre (212.132, 150) ccw
  line L898 (161.0254, 180.2798) -> (159.6217, 181.1115)
  arc A17 (236.3452, 217.2191) -> (232.0535, 218.6136) centre (212.132, 150) ccw
  arc A18 (236.3452, 217.2191) -> (232.0535, 218.6136) centre (212.132, 150) ccw